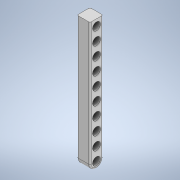
# Autodesk Inventor part: Stang3D
Saved by Autodesk Inventor 2022 (Build 260153000, 153)
## iProperties
Created: 2022-04-10
Part Number: Stang3D
Material: Generic
Document SubType Name: Modeling
Designer: Patrick
Density: 1 g/cm^3
Appearance: Default
Author: Patrick
Autodesk Inventor part; units mm, degrees
ref_plane "YZ Plane" through (0, 0, 0) normal (1, 0, 0) x (0, 1, 0)
ref_plane "XZ Plane" through (0, 0, 0) normal (0, 1, 0) x (-1, 0, 0)
ref_plane "XY Plane" through (0, 0, 0) normal (0, 0, 1) x (1, 0, 0)
sketch "Sketch1" plane through (0, 0, 0) normal (0, 1, 0) x (-1, 0, 0)
  line L0 (0, 0) -> (10, 0)
  line L1 (10, 0) -> (10, -10)
  line L2 (10, -10) -> (0, -10)
  line L3 (0, -10) -> (0, 0)
  dimension "d0" = 10
  dimension "d1" = 10
  constraints: 8 end point, 2 parallel, 1 horizontal, 1 perpendicular
  measures "d0" distance of L1.end L2.end
  measures "d1" distance of L2.end L0.start
extrude "Extrusion1" add sketch "Sketch1" along normal blind 100
sketch "Sketch2" plane through (0, 0, 0) normal (1, 0, 0) x (0, 0, -1)
  circle A0 centre (5, 95) radius 3
  line L0 (10, 0) -> (10, 100) projected
  line L1 (0, 100) -> (10, 100) projected
  line L2 (0, 0) -> (10, 0) projected
  line L3 (10, 0) -> (10, 100) projected
  line L4 (0, 100) -> (10, 100) projected
  line L5 (0, 0) -> (0, 100) projected
  circle A1 centre (5, 85) radius 3
  circle A2 centre (5, 75) radius 3
  circle A3 centre (5, 65) radius 3
  circle A4 centre (5, 55) radius 3
  circle A5 centre (5, 45) radius 3
  circle A6 centre (5, 35) radius 3
  circle A7 centre (5, 25) radius 3
  circle A8 centre (5, 15) radius 3
  circle A9 centre (5, 5) radius 3
  line L6 (0, 0) -> (0, 100) projected
  line L7 (10, 0) -> (10, 100) projected
  arc A10 (0, 5) -> (10, 5) centre (5, 5) ccw
  line L8 (10, 0) -> (0, 0) projected
  point P0 (5, 0)
  point P1 (0, 5)
  point P2 (10, 5)
  dimension "d4" = 6
  dimension "d5" = 5
  dimension "d6" = 5
  dimension "d9" = 10
  constraints: 11 centre point, 2 point on circle, 2 point on line, 1 tangent, 1 vertical, 18 other
  measures "d4" diameter of A0
  measures "d5" distance from line of L0 A0.centre
  measures "d6" distance from line of L1 A0.centre
  measures "d9" distance of A0.centre A1.centre
extrude "Extrusion2" cut sketch "Sketch2" against normal through all contours A0 | L2 A10 L0 | L2 L5 A10 | A1 | A2 | A3 | A4 | A5 | A6 | A7 | A8 | A9
fillet "Fillet1" radius 1 6 edges at (0, 0, -5) (0, 52.5, -10) (0, 52.5, 0) (-10, 0, -5) (-10, 52.5, -10) (-10, 52.5, 0)
body "Solid1"
